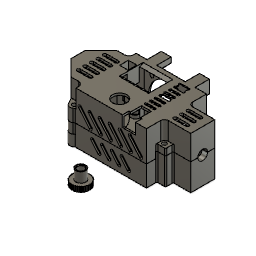
Case_Car_Bat_Mount_Spot Welder_V3 (Autodesk Fusion 360 design; units mm, degrees)
Autodesk Fusion 360 part; units mm, degrees
(part 1 of 5)
sketch "Skizze1" plane through (0, 0, 0) normal (0, 1, 0) x (1, 0, 0)
  circle A0 centre (-27, 22) radius 1.9
  line L0 (1.75, 0) -> (22.5, 0)
  line L1 (0, -1.75) -> (0, -22.5)
  circle A1 centre (27, 22) radius 1.9
  circle A2 centre (-27, -22) radius 1.9
  circle A3 centre (27, -22) radius 1.9
  line L2 (-32.5, 27.5) -> (32.5, 27.5)
  line L3 (32.5, 27.5) -> (32.5, -27.5)
  line L4 (32.5, -27.5) -> (-32.5, -27.5)
  line L5 (-32.5, -27.5) -> (-32.5, 27.5)
  line L6 (-32.5, 27.5) -> (32.5, -27.5) construction
  line L7 (32.5, 27.5) -> (-32.5, -27.5) construction
  point P0 (51.5, 9.5)
  dimension "d3" = 3.8
  dimension "d9" = 22
  dimension "d10" = 27
  dimension "d11" = 65
  dimension "d12" = 55
  constraint symmetric A0 L1 A1
  constraint symmetric A0 L0 A2
  constraint symmetric L0 A1 A3
  constraint perpendicular L2 L3
  constraint parallel L2 L4
  constraint parallel L3 L5
  constraint horizontal L2
  constraint coincident L6 origin
  constraint coincident L7 origin
  measures "d3" diameter of A0
  measures "d9" distance of A0.centre L0
  measures "d10" distance of A0.centre L1
  measures "d11" distance of L3.end L4.end
  measures "d12" distance of L2.end L3.end
extrude "Extrusion1" add sketch "Skizze1" along normal blind 3 makes body 1
sketch "Skizze2" plane through (0, 0, 0) normal (0, -1, 0) x (1, 0, 0)
  circle A0 centre (-27, 22) radius 1.9
  circle A1 centre (-27, -22) radius 1.9
  circle A2 centre (27, 22) radius 1.9
  circle A3 centre (27, -22) radius 1.9
  line L0 (32.5, 27.5) -> (-32.5, 27.5)
  line L1 (-32.5, 27.5) -> (-32.5, -27.5)
  line L2 (-32.5, -27.5) -> (32.5, -27.5)
  line L3 (32.5, -27.5) -> (32.5, 27.5)
  circle A4 centre (-27, 22) radius 1.9
  circle A5 centre (-27, -22) radius 1.9
  circle A6 centre (27, 22) radius 1.9
  circle A7 centre (27, -22) radius 1.9
  line L4 (-32.5, 27.5) -> (32.5, 27.5)
  line L5 (32.5, 27.5) -> (32.5, -27.5)
  line L6 (32.5, -27.5) -> (-32.5, -27.5)
  line L7 (-32.5, -27.5) -> (-32.5, 27.5)
extrude "Extrusion2" add sketch "Skizze2" against normal blind 1.5 contours A0 A4 | A1 A5 | A2 A6 | A3 A7 bodies 1
sketch "Skizze3" plane through (0, 3, 0) normal (0, 1, 0) x (-1, 0, 0)
  circle A0 centre (27, 22) radius 1.9
  circle A1 centre (27, -22) radius 1.9
  circle A2 centre (-27, 22) radius 1.9
  circle A3 centre (-27, -22) radius 1.9
  line L0 (32.5, 27.5) -> (-32.5, 27.5)
  line L1 (-32.5, 27.5) -> (-32.5, -27.5)
  line L2 (-32.5, -27.5) -> (32.5, -27.5)
  line L3 (32.5, -27.5) -> (32.5, 27.5)
  circle A4 centre (27, -22) radius 4
  circle A5 centre (-27, -22) radius 4
  circle A6 centre (27, 22) radius 4
  circle A7 centre (-27, 22) radius 4
  dimension "d17" = 8
  dimension "d18" = 8
  dimension "d19" = 8
  dimension "d20" = 8
  constraint concentric A1 A4
  constraint concentric A3 A5
  constraint concentric A0 A6
  constraint concentric A2 A7
  measures "d17" diameter of A4
  measures "d18" diameter of A6
  measures "d19" diameter of A7
  measures "d20" diameter of A5
extrude "Extrusion3" add sketch "Skizze3" along normal blind 3 contours A4 | A5 | A6 | A7 bodies 1
sketch "Skizze4" plane through (0, 6, 0) normal (0, 1, 0) x (-1, 0, 0)
  circle A0 centre (27, -22) radius 1.9
  circle A1 centre (27, -22) radius 4
  circle A2 centre (27, -22) radius 3
  circle A3 centre (-27, -22) radius 1.9
  circle A4 centre (-27, 22) radius 1.9
  circle A5 centre (27, 22) radius 1.9
  circle A6 centre (-27, -22) radius 3
  circle A7 centre (-27, 22) radius 3
  circle A8 centre (27, 22) radius 3
  dimension "d23" = 6
  dimension "d24" = 6
  dimension "d25" = 6
  dimension "d26" = 6
  constraint concentric A0 A2
  constraint concentric A3 A6
  constraint concentric A4 A7
  constraint concentric A5 A8
  measures "d23" diameter of A2
  measures "d24" diameter of A8
  measures "d25" diameter of A7
  measures "d26" diameter of A6
extrude "Extrusion4" add sketch "Skizze4" along normal blind 4 contours A2 | A6 | A7 | A8 bodies 1
sketch "Skizze5" plane through (0, 0, 0) normal (0, -1, 0) x (1, 0, 0)
  line L0 (32.5, 27.5) -> (-32.5, 27.5)
  line L1 (-32.5, 27.5) -> (-32.5, -27.5)
  line L2 (-32.5, -27.5) -> (32.5, -27.5)
  line L3 (32.5, -27.5) -> (32.5, 27.5)
  line L4 (32.5, -11) -> (56.5, -11)
  line L5 (56.5, -11) -> (56.5, 11)
  line L6 (56.5, 11) -> (32.5, 11)
  line L7 (32.5, 11) -> (32.5, -11)
  line L8 (1.75, 0) -> (22.5, 0)
  dimension "d29" = 24
  dimension "d31" = 22
  constraint horizontal L4
  constraint vertical L5
  constraint horizontal L6
  constraint vertical L7
  constraint coincident L3 L4.start
  constraint symmetric L4 L6 L8
  measures "d29" distance of L4.start L4.end
  measures "d31" vertical distance of L4.end L5.end
extrude "Extrusion5" add sketch "Skizze5" against normal blind 3 contours L3 L4 L5 L6 L7 bodies 1
sketch "Skizze6" plane through (0, 0, 0) normal (0, -1, 0) x (1, 0, 0)
  line L0 (32.5, 27.5) -> (-32.5, 27.5)
  line L1 (-32.5, 27.5) -> (-32.5, -27.5)
  line L2 (-32.5, -27.5) -> (32.5, -27.5)
  line L3 (32.5, -27.5) -> (32.5, -11)
  line L4 (32.5, -11) -> (56.5, -11)
  line L5 (56.5, -11) -> (56.5, 11)
  line L6 (56.5, 11) -> (32.5, 11)
  line L7 (32.5, 11) -> (32.5, 27.5)
  line L8 (-32.5, -21.5) -> (-42.5, -21.5)
  line L9 (-42.5, -21.5) -> (-42.5, 21.5)
  line L10 (-42.5, 21.5) -> (-32.5, 21.5)
  line L11 (-32.5, 21.5) -> (-32.5, -21.5)
  line L12 (1.75, 0) -> (22.5, 0)
  line L13 (-42.5, -21.5) -> (-57.5, -6.5)
  line L14 (-42.5, -21.5) -> (-24.6723, -21.5) construction
  line L15 (-42.5, 21.5) -> (-57.5, 6.5)
  line L16 (-42.5, 21.5) -> (-24.5, 21.5) construction
  line L17 (-57.5, 6.5) -> (-57.5, -6.5)
  dimension "d34" = 10
  dimension "d35" = 43
  dimension "d36" = 135
  dimension "d37" = 135
  dimension "d38" = 15
  constraint horizontal L8
  constraint vertical L9
  constraint horizontal L10
  constraint vertical L11
  constraint coincident L1 L8.start
  constraint symmetric L8 L10 L12
  constraint horizontal L14
  constraint horizontal L16
  constraint parallel L9 L17
  measures "d34" distance of L8.start L8.end
  measures "d35" distance of L8.start L10.end
  measures "d36" angle of L13 L14
  measures "d37" angle of L15 L16
  measures "d38" distance of L9 L17
extrude "Extrusion6" add sketch "Skizze6" against normal blind 3 contours L1 L8 L9 L10 L11 | L9 L13 L15 L17 bodies 1
sketch "Skizze7" plane through (0, 3, 0) normal (0, 1, 0) x (-1, 0, 0)
  circle A0 centre (-27, -22) radius 4
  circle A1 centre (27, -22) radius 4
  circle A2 centre (-27, 22) radius 4
  circle A3 centre (27, 22) radius 4
  line L0 (32.5, 27.5) -> (-32.5, 27.5)
  line L1 (-32.5, 27.5) -> (-32.5, 11)
  line L2 (-32.5, 11) -> (-56.5, 11)
  line L3 (-56.5, 11) -> (-56.5, -11)
  line L4 (-56.5, -11) -> (-32.5, -11)
  line L5 (-32.5, -11) -> (-32.5, -27.5)
  line L6 (-32.5, -27.5) -> (32.5, -27.5)
  line L7 (32.5, -27.5) -> (32.5, -21.5)
  line L8 (32.5, -21.5) -> (42.5, -21.5)
  line L9 (42.5, -21.5) -> (57.5, -6.5)
  line L10 (57.5, -6.5) -> (57.5, 6.5)
  line L11 (57.5, 6.5) -> (42.5, 21.5)
  line L12 (42.5, 21.5) -> (32.5, 21.5)
  line L13 (32.5, 21.5) -> (32.5, 27.5)
  line L14 (32.5, -27.5) -> (32.5, -21.5)
  line L15 (-32.5, -27.5) -> (32.5, -27.5)
  line L16 (32.5, -21.5) -> (42.5, -21.5)
  line L17 (42.5, -21.5) -> (57.5, -6.5)
  line L18 (57.5, -6.5) -> (57.5, 6.5)
  line L19 (57.5, 6.5) -> (42.5, 21.5)
  line L20 (42.5, 21.5) -> (32.5, 21.5)
  line L21 (32.5, 21.5) -> (32.5, 27.5)
  line L22 (32.5, 27.5) -> (-32.5, 27.5)
  line L23 (-32.5, 27.5) -> (-32.5, 11)
  line L24 (-32.5, 11) -> (-56.5, 11)
  line L25 (-32.5, 27.5) -> (32.5, 27.5)
  line L26 (32.5, 27.5) -> (32.5, 21.5)
  line L27 (32.5, 21.5) -> (42.5, 21.5)
  line L28 (42.5, 21.5) -> (57.5, 6.5)
  line L29 (57.5, 6.5) -> (57.5, -6.5)
  line L30 (57.5, -6.5) -> (42.5, -21.5)
  line L31 (42.5, -21.5) -> (32.5, -21.5)
  line L32 (32.5, -21.5) -> (32.5, -27.5)
  line L33 (32.5, -27.5) -> (-32.5, -27.5)
  line L34 (-32.5, -27.5) -> (-32.5, -11)
  line L35 (-32.5, -11) -> (-56.5, -11)
  line L36 (-56.5, -11) -> (-56.5, 11)
  line L37 (-56.5, 11) -> (-32.5, 11)
  line L38 (-32.5, 11) -> (-32.5, 27.5)
  line L39 (31, -26) -> (-31, -26)
  line L40 (-31, -26) -> (-31, -9.8787)
  line L41 (-31, -9.8787) -> (-31, -9.5)
  line L42 (-31, -9.5) -> (-55, -9.5)
  line L43 (-55, -9.5) -> (-55, 9.5)
  line L44 (-55, 9.5) -> (-31, 9.5)
  line L45 (-31, 9.5) -> (-31, 26)
  line L46 (-31, 26) -> (31, 26)
  line L47 (31, 26) -> (31, 20)
  line L48 (31, 20) -> (41.8787, 20)
  line L49 (41.8787, 20) -> (56, 5.8787)
  line L50 (56, 5.8787) -> (56, -5.8787)
  line L51 (56, -5.8787) -> (41.8787, -20)
  line L52 (41.8787, -20) -> (31, -20)
  line L53 (31, -20) -> (31, -26)
  dimension "d41" = 1.5
  dimension "d42" = 1.5
  dimension "d43" = 1.5
  dimension "d44" = 1.5
  dimension "d45" = 1.5
  dimension "d46" = 1.5
  dimension "d47" = 1.5
  dimension "d48" = 1.5
  dimension "d49" = 1.5
  dimension "d50" = 1.5
  dimension "d51" = 1.5
  dimension "d52" = 1.5
  dimension "d53" = 1.5
  dimension "d54" = 1.5
  constraint perpendicular L7 L39
  constraint perpendicular L35 L40
  constraint perpendicular L35 L41
  constraint perpendicular L40 L42
  constraint perpendicular L42 L43
  constraint perpendicular L43 L44
  constraint perpendicular L44 L45
  constraint perpendicular L26 L46
  constraint perpendicular L46 L47
  constraint perpendicular L47 L48
  constraint perpendicular L46 L50
  constraint perpendicular L50 L52
  constraint perpendicular L39 L53
  constraint parallel L9 L51
  constraint parallel L11 L49
  measures "d41" distance of L10 L50
  measures "d42" distance of L9 L51
  measures "d43" distance of L8 L52
  measures "d44" distance of L7 L53
  measures "d45" distance of L6 L39
  measures "d46" distance of L5 L40
  measures "d47" distance of L4 L42
  measures "d48" distance of L3 L43
  measures "d49" distance of L2 L44
  measures "d50" distance of L1 L45
  measures "d51" distance of L0 L46
  measures "d52" distance of L13 L47
  measures "d53" distance of L12 L48
  measures "d54" distance of L11 L49
extrude "Extrusion7" add sketch "Skizze7" along normal blind 13 bodies 1
sketch "Skizze8" plane through (0, 3, 0) normal (0, 1, 0) x (-1, 0, 0)
  line L0 (51.5218, -10.3569) -> (51.5218, 10.3569)
  line L1 (-31, -9.5) -> (-31, -22)
  line L2 (-31, 22) -> (-31, 9.5)
  line L3 (-31, 9.5) -> (-55, 9.5)
  line L4 (-55, 9.5) -> (-55, -9.5)
  line L5 (-55, -9.5) -> (-31, -9.5)
  line L6 (-27, -26) -> (27, -26)
  arc A0 (31, -22) -> (27, -26) centre (27, -22) ccw
  line L7 (31, -22) -> (31, -20)
  line L8 (31, -20) -> (41.8787, -20)
  line L9 (41.8787, -20) -> (56, -5.8787)
  line L10 (56, -5.8787) -> (56, 5.8787)
  line L11 (56, 5.8787) -> (41.8787, 20)
  line L12 (41.8787, 20) -> (31, 20)
  line L13 (31, 20) -> (31, 22)
  arc A1 (27, 26) -> (31, 22) centre (27, 22) ccw
  arc A2 (-31, 22) -> (-27, 26) centre (-27, 22) ccw
  line L14 (27, 26) -> (-27, 26)
  arc A3 (-27, -26) -> (-31, -22) centre (-27, -22) ccw
  constraint coincident L0.end L11
  constraint coincident L0.start L9
  constraint parallel L0 L10
extrude "Extrusion8" add sketch "Skizze8" along normal up to surface (13 mm away) contours L0 L9 L10 L11 bodies 1
sketch "Skizze9" plane through (-57.5, 0, 0) normal (-1, 0, 0) x (0, 0, 1)
  line L0 (-6.5, 0) -> (6.5, 0)
  line L1 (6.5, 0) -> (6.5, 16)
  line L2 (6.5, 16) -> (-6.5, 16)
  line L3 (-6.5, 16) -> (-6.5, 0)
  line L4 (0, 1.75) -> (0, 22.5)
  line L5 (-6.5, 16) -> (6.5, 16)
  circle A0 centre (0, 16) radius 5
  dimension "d60" = 10
  constraint midpoint L5 A0.centre
  measures "d60" diameter of A0
extrude "Extrusion9" cut sketch "Skizze9" against normal blind 6 contours L2 L4 L5 A0 | L2 L4 L5 A0 picked at (-3.3164, 15.7628) picked at (2.6617, 14.0075) bodies 1
sketch "Skizze12" plane through (0, 3, 0) normal (0, 1, 0) x (-1, 0, 0)
  line L0 (51.5218, -10.3569) -> (51.5218, 10.3569)
  line L1 (51.5218, 10.3569) -> (41.8787, 20)
  line L2 (41.8787, 20) -> (31, 20)
  line L3 (31, 20) -> (31, 22)
  arc A0 (27, 26) -> (31, 22) centre (27, 22) ccw
  arc A1 (-31, 22) -> (-27, 26) centre (-27, 22) ccw
  line L4 (-31, 22) -> (-31, 9.5)
  line L5 (-31, 9.5) -> (-55, 9.5)
  line L6 (-55, 9.5) -> (-55, -9.5)
  line L7 (-55, -9.5) -> (-31, -9.5)
  arc A2 (-27, -26) -> (-31, -22) centre (-27, -22) ccw
  arc A3 (31, -22) -> (27, -26) centre (27, -22) ccw
  line L8 (31, -22) -> (31, -20)
  line L9 (31, -20) -> (41.8787, -20)
  line L10 (41.8787, -20) -> (51.5218, -10.3569)
  line L11 (-51.5, 9.5) -> (-51.5, -9.5)
  line L12 (-31, -9.5) -> (-31, -22)
  line L13 (-27, -26) -> (27, -26)
  line L14 (27, 26) -> (-27, 26)
  constraint coincident L5 L11.start
  constraint coincident L7 L11.end
  constraint parallel L6 L11
extrude "Extrusion12" add sketch "Skizze12" along normal blind 13 contours L5 L6 L7 L11 bodies 1
sketch "Skizze16" plane through (0, 6, 0) normal (0, 1, 0) x (-1, 0, 0)
  circle A0 centre (27, -22) radius 3
  line L0 (-51.5, 9.5) -> (-51.5, -9.5)
  line L1 (-51.5, -9.5) -> (-31, -9.5)
  line L2 (-31, -9.5) -> (-31, -22)
  arc A1 (-27, -26) -> (-31, -22) centre (-27, -22) ccw
  line L3 (-27, -26) -> (27, -26)
  arc A2 (31, -22) -> (27, -26) centre (27, -22) ccw
  line L4 (31, -22) -> (31, -20)
  line L5 (31, -20) -> (41.8787, -20)
  line L6 (41.8787, -20) -> (51.5218, -10.3569)
  line L7 (51.5218, -10.3569) -> (51.5218, 10.3569)
  line L8 (51.5218, 10.3569) -> (41.8787, 20)
  line L9 (41.8787, 20) -> (31, 20)
  line L10 (31, 20) -> (31, 22)
  arc A3 (27, 26) -> (31, 22) centre (27, 22) ccw
  line L11 (27, 26) -> (-27, 26)
  arc A4 (-31, 22) -> (-27, 26) centre (-27, 22) ccw
  line L12 (-31, 22) -> (-31, 9.5)
  line L13 (-31, 9.5) -> (-51.5, 9.5)
  line L14 (31, -22) -> (23, -22)
  line L15 (23, -22) -> (23, -26)
  line L16 (23, -26) -> (31, -26)
  line L17 (31, -26) -> (31, -22)
  line L18 (-31, -26) -> (-23, -26)
  line L19 (-23, -26) -> (-23, -22)
  line L20 (-23, -22) -> (-31, -22)
  line L21 (-31, -22) -> (-31, -26)
  line L22 (-31, 22) -> (-23, 22)
  line L23 (-23, 22) -> (-23, 26)
  line L24 (-23, 26) -> (-31, 26)
  line L25 (-31, 26) -> (-31, 22)
  line L26 (31, 22) -> (23, 22)
  line L27 (23, 22) -> (23, 26)
  line L28 (23, 26) -> (31, 26)
  line L29 (31, 26) -> (31, 22)
  circle A5 centre (27, 22) radius 1.9
  circle A6 centre (27, 22) radius 3
  circle A7 centre (27, -22) radius 1.9
  circle A8 centre (27, -22) radius 1.9
  circle A9 centre (27, -22) radius 3
  circle A10 centre (-27, -22) radius 1.9
  circle A11 centre (-27, -22) radius 3
  circle A12 centre (-27, 22) radius 1.9
  circle A13 centre (-27, 22) radius 3
  arc A14 (31, -22) -> (27, -26) centre (27, -22) ccw
  arc A15 (27, -26) -> (31, -22) centre (27, -22) ccw
  point P0 (-31, -26)
  dimension "d76" = 4
  dimension "d77" = 8
  dimension "d78" = 8
  dimension "d79" = 8
  constraint horizontal L14
  constraint vertical L15
  constraint horizontal L16
  constraint vertical L17
  constraint coincident A2.start L4.start
  constraint horizontal L18
  constraint vertical L19
  constraint horizontal L20
  constraint vertical L21
  constraint coincident P0 L18.start
  constraint horizontal L22
  constraint vertical L23
  constraint horizontal L24
  constraint vertical L25
  constraint coincident A4.start L12.start
  constraint horizontal L26
  constraint vertical L27
  constraint horizontal L28
  constraint vertical L29
  constraint coincident L10.end A3.end
  measures "d76" distance of P0 L2.end
  measures "d77" distance of P0 L18.end
  measures "d78" distance of A4.start L22.end
  measures "d79" distance of L10.end L26.end
extrude "Extrusion15" add sketch "Skizze16" along normal blind 4 and the other way blind 3 contours A0 A2 L14 A9 A14 A15 | L16 L17 A15 | L3 A2 L15 L16 A14 | A1 L3 L18 L19 | A1 L18 L20 L21 A11 | A3 L26 L28 L29 A6 | A3 L11 L27 L28 | A4 L22 L24 L25 A13 | L11 A4 L23 L24 bodies 1
sketch "Skizze18" plane through (0, 3, 0) normal (0, 1, 0) x (-1, 0, 0)
  line L0 (-23, 26) -> (-23, 22)
  arc A0 (-31, 22) -> (-23, 22) centre (-27, 22) ccw
  line L1 (-31, 22) -> (-31, 9.5)
  line L2 (-31, 9.5) -> (-51.5, 9.5)
  line L3 (-51.5, 9.5) -> (-51.5, -9.5)
  line L4 (-51.5, -9.5) -> (-31, -9.5)
  line L5 (-31, -9.5) -> (-31, -22)
  arc A1 (-23, -22) -> (-31, -22) centre (-27, -22) ccw
  line L6 (-23, -22) -> (-23, -26)
  line L7 (-23, -26) -> (23, -26)
  line L8 (23, -26) -> (23, -22)
  arc A2 (31, -22) -> (23, -22) centre (27, -22) ccw
  line L9 (31, -22) -> (31, -20)
  line L10 (31, -20) -> (41.8787, -20)
  line L11 (41.8787, -20) -> (51.5218, -10.3569)
  line L12 (51.5218, -10.3569) -> (51.5218, 10.3569)
  line L13 (51.5218, 10.3569) -> (41.8787, 20)
  line L14 (41.8787, 20) -> (31, 20)
  line L15 (31, 20) -> (31, 22)
  arc A3 (23, 22) -> (31, 22) centre (27, 22) ccw
  line L16 (23, 22) -> (23, 26)
  line L17 (23, 26) -> (-23, 26)
  circle A4 centre (36, 25) radius 3.5
  line L18 (32.5, 21.5) -> (32.5, 27.5)
  line L19 (42.5, 21.5) -> (32.5, 21.5)
  circle A5 centre (36, 25) radius 1.9
  line L20 (42.5, 21.5) -> (38.922, 26.9266)
  line L21 (32.5, 27.5) -> (34.8649, 28.3108)
  line L22 (-1.75, 0) -> (-22.5, 0)
  line L23 (42.5, -21.5) -> (38.922, -26.9266)
  circle A6 centre (36, -25) radius 3.5
  line L24 (32.5, -27.5) -> (34.8649, -28.3108)
  circle A7 centre (36, -25) radius 1.9
  line L25 (42.5, -21.5) -> (32.5, -21.5)
  line L26 (32.5, -21.5) -> (32.5, -27.5)
  dimension "d89" = 7
  dimension "d90" = 3.8
  constraint tangent A4 L18
  constraint tangent A4 L19
  constraint concentric A4 A5
  constraint coincident L19.start L20.start
  constraint coincident A4 L20.end
  constraint tangent A4 L20
  constraint coincident L18.end L21.start
  constraint coincident A4 L21.end
  constraint tangent A4 L21
  constraint symmetric A4 L22 A6
  constraint symmetric L18.start L22 L25.end
  constraint symmetric L18.end L22 L24.start
  constraint symmetric L19.start L22 L23.start
  constraint symmetric A5 L22 A7
  constraint symmetric L20.end L22 L23.end
  constraint symmetric L21.end L22 L24.end
  measures "d89" diameter of A4
  measures "d90" diameter of A5
extrude "Extrusion16" add sketch "Skizze18" along normal blind 13 and the other way blind 3 contours A4 | A4 L19 L20 | A4 L18 L19 | A4 L18 L21 | L23 A6 L25 | A6 | A6 L25 L26 | A6 L24 L26 bodies 1
sketch "Skizze19" plane through (0, 3, 0) normal (0, 1, 0) x (-1, 0, 0)
  line L0 (-23, 26) -> (-23, 22)
  arc A0 (-31, 22) -> (-23, 22) centre (-27, 22) ccw
  line L1 (-31, 22) -> (-31, 9.5)
  line L2 (-31, 9.5) -> (-51.5, 9.5)
  line L3 (-51.5, 9.5) -> (-51.5, -9.5)
  line L4 (-51.5, -9.5) -> (-31, -9.5)
  line L5 (-31, -9.5) -> (-31, -22)
  arc A1 (-23, -22) -> (-31, -22) centre (-27, -22) ccw
  line L6 (-23, -22) -> (-23, -26)
  line L7 (-23, -26) -> (23, -26)
  line L8 (23, -26) -> (23, -22)
  arc A2 (31, -22) -> (23, -22) centre (27, -22) ccw
  line L9 (31, -22) -> (31, -20)
  line L10 (31, -20) -> (41.8787, -20)
  line L11 (41.8787, -20) -> (51.5218, -10.3569)
  line L12 (51.5218, -10.3569) -> (51.5218, 10.3569)
  line L13 (51.5218, 10.3569) -> (41.8787, 20)
  line L14 (41.8787, 20) -> (31, 20)
  line L15 (31, 20) -> (31, 22)
  arc A3 (23, 22) -> (31, 22) centre (27, 22) ccw
  line L16 (23, 22) -> (23, 26)
  line L17 (23, 26) -> (-23, 26)
  line L18 (-32.5, 11) -> (-39.5, 11)
  line L19 (-39.5, 11) -> (-39.5, 18)
  line L20 (-39.5, 18) -> (-32.5, 18)
  line L21 (-32.5, 18) -> (-32.5, 11)
  circle A4 centre (-36, 14.5) radius 1.9
  line L22 (-1.75, 0) -> (-22.5, 0)
  line L23 (-39.5, -11) -> (-39.5, -18)
  line L24 (-39.5, -18) -> (-32.5, -18)
  circle A5 centre (-36, -14.5) radius 1.9
  line L25 (-32.5, -11) -> (-32.5, -27.5)
  line L26 (-56.5, -11) -> (-32.5, -11)
  point P0 (-32.5, 11)
  dimension "d95" = 7
  dimension "d96" = 7
  dimension "d97" = 3.8
  dimension "d98" = 3.5
  dimension "d99" = 3.5
  constraint horizontal L18
  constraint vertical L19
  constraint horizontal L20
  constraint vertical L21
  constraint coincident P0 L18.start
  constraint symmetric L18.end L22 L23.start
  constraint symmetric L19.end L22 L23.end
  constraint symmetric L20.end L22 L24.end
  constraint symmetric A4 L22 A5
  measures "d95" distance of P0 L18.end
  measures "d96" distance of P0 L20.end
  measures "d97" diameter of A4
  measures "d98" distance of L18 A4.centre
  measures "d99" distance of L21 A4.centre
extrude "Extrusion17" add sketch "Skizze19" along normal blind 13 and the other way blind 3 contours L18 L19 L20 L21 | L23 L24 L25 L26 bodies 1
fillet "Abrundung1" radius 1 6 edges at (32.5, 8, 18) (39.5, 8, 11) (39.5, 8, -11) (32.5, 8, -18) (39.5, 8, 18) (39.5, 8, -18) on bodies 1
sketch "Skizze20" plane through (0, 16, 0) normal (0, 1, 0) x (-1, 0, 0)
  arc A0 (-39.5, -17) -> (-38.5, -18) centre (-38.5, -17) ccw
  line L0 (-38.5, -18) -> (-33.5, -18)
  arc A1 (-32.5, -19) -> (-33.5, -18) centre (-33.5, -19) ccw
  line L1 (-32.5, -19) -> (-32.5, -27.5)
  line L2 (-32.5, -27.5) -> (32.5, -27.5)
  line L3 (32.5, -27.5) -> (34.8649, -28.3108)
  arc A2 (34.8649, -28.3108) -> (38.922, -26.9266) centre (36, -25) ccw
  line L4 (38.922, -26.9266) -> (42.5, -21.5)
  line L5 (42.5, -21.5) -> (57.5, -6.5)
  line L6 (57.5, -6.5) -> (57.5, -5)
  line L7 (57.5, -5) -> (51.5218, -5)
  line L8 (51.5218, -5) -> (51.5218, -10.3569)
  line L9 (51.5218, -10.3569) -> (41.8787, -20)
  line L10 (41.8787, -20) -> (31, -20)
  line L11 (31, -20) -> (31, -26)
  line L12 (31, -26) -> (-31, -26)
  line L13 (-31, -26) -> (-31, -9.5)
  line L14 (-31, -9.5) -> (-51.5, -9.5)
  line L15 (-51.5, -9.5) -> (-51.5, 9.5)
  line L16 (-51.5, 9.5) -> (-31, 9.5)
  line L17 (-31, 9.5) -> (-31, 26)
  line L18 (-31, 26) -> (31, 26)
  line L19 (31, 26) -> (31, 20)
  line L20 (31, 20) -> (41.8787, 20)
  line L21 (41.8787, 20) -> (51.5218, 10.3569)
  line L22 (51.5218, 10.3569) -> (51.5218, 5)
  line L23 (51.5218, 5) -> (57.5, 5)
  line L24 (57.5, 5) -> (57.5, 6.5)
  line L25 (57.5, 6.5) -> (42.5, 21.5)
  line L26 (42.5, 21.5) -> (38.922, 26.9266)
  arc A3 (38.922, 26.9266) -> (34.8649, 28.3108) centre (36, 25) ccw
  line L27 (34.8649, 28.3108) -> (32.5, 27.5)
  line L28 (32.5, 27.5) -> (-32.5, 27.5)
  line L29 (-32.5, 27.5) -> (-32.5, 19)
  arc A4 (-33.5, 18) -> (-32.5, 19) centre (-33.5, 19) ccw
  line L30 (-33.5, 18) -> (-38.5, 18)
  arc A5 (-38.5, 18) -> (-39.5, 17) centre (-38.5, 17) ccw
  line L31 (-39.5, 17) -> (-39.5, 12)
  arc A6 (-40.5, 11) -> (-39.5, 12) centre (-40.5, 12) ccw
  line L32 (-40.5, 11) -> (-56.5, 11)
  line L33 (-56.5, 11) -> (-56.5, -11)
  line L34 (-56.5, -11) -> (-40.5, -11)
  arc A7 (-39.5, -12) -> (-40.5, -11) centre (-40.5, -12) ccw
  line L35 (-39.5, -12) -> (-39.5, -17)
  circle A8 centre (-36, 14.5) radius 1.9
  circle A9 centre (-36, -14.5) radius 1.9
  circle A10 centre (36, -25) radius 1.9
  circle A11 centre (36, 25) radius 1.9
  circle A12 centre (-36, 14.5) radius 1.9
  circle A13 centre (-36, -14.5) radius 1.9
  circle A14 centre (36, -25) radius 1.9
  circle A15 centre (36, 25) radius 1.9
  arc A16 (-39.5, -17) -> (-38.5, -18) centre (-38.5, -17) ccw
  line L36 (-39.5, -17) -> (-39.5, -12)
  arc A17 (-39.5, -12) -> (-40.5, -11) centre (-40.5, -12) ccw
  line L37 (-40.5, -11) -> (-56.5, -11)
  line L38 (-56.5, -11) -> (-56.5, 11)
  line L39 (-56.5, 11) -> (-40.5, 11)
  arc A18 (-40.5, 11) -> (-39.5, 12) centre (-40.5, 12) ccw
  line L40 (-39.5, 12) -> (-39.5, 17)
  arc A19 (-38.5, 18) -> (-39.5, 17) centre (-38.5, 17) ccw
  line L41 (-38.5, 18) -> (-33.5, 18)
  arc A20 (-33.5, 18) -> (-32.5, 19) centre (-33.5, 19) ccw
  line L42 (-32.5, 19) -> (-32.5, 27.5)
  line L43 (-32.5, 27.5) -> (32.5, 27.5)
  line L44 (32.5, 27.5) -> (34.8649, 28.3108)
  arc A21 (38.922, 26.9266) -> (34.8649, 28.3108) centre (36, 25) ccw
  line L45 (38.922, 26.9266) -> (42.5, 21.5)
  line L46 (42.5, 21.5) -> (57.5, 6.5)
  line L47 (57.5, 6.5) -> (57.5, -6.5)
  line L48 (57.5, -6.5) -> (42.5, -21.5)
  line L49 (42.5, -21.5) -> (38.922, -26.9266)
  arc A22 (34.8649, -28.3108) -> (38.922, -26.9266) centre (36, -25) ccw
  line L50 (34.8649, -28.3108) -> (32.5, -27.5)
  line L51 (32.5, -27.5) -> (-32.5, -27.5)
  line L52 (-32.5, -27.5) -> (-32.5, -19)
  arc A23 (-32.5, -19) -> (-33.5, -18) centre (-33.5, -19) ccw
  line L53 (-33.5, -18) -> (-38.5, -18)
  line L54 (-51.5, -9.5) -> (-51.5, 9.5)
  line L55 (-51.5, 9.5) -> (-31, 9.5)
  line L56 (-23, 26) -> (-23, 22)
  arc A24 (-31, 22) -> (-23, 22) centre (-27, 22) ccw
  line L57 (-31, 22) -> (-31, 9.5)
  line L58 (-31, 9.5) -> (-51.5, 9.5)
  line L59 (-51.5, 9.5) -> (-51.5, -9.5)
  line L60 (-51.5, -9.5) -> (-31, -9.5)
  line L61 (-31, -9.5) -> (-31, -22)
  arc A25 (-23, -22) -> (-31, -22) centre (-27, -22) ccw
  line L62 (-23, -22) -> (-23, -26)
  line L63 (-23, -26) -> (23, -26)
  line L64 (23, -26) -> (23, -22)
  arc A26 (31, -22) -> (23, -22) centre (27, -22) ccw
  line L65 (31, -22) -> (31, -20)
  line L66 (31, -20) -> (41.8787, -20)
  line L67 (41.8787, -20) -> (51.5218, -10.3569)
  line L68 (51.5218, -10.3569) -> (51.5218, 10.3569)
  line L69 (51.5218, 10.3569) -> (41.8787, 20)
  line L70 (41.8787, 20) -> (31, 20)
  line L71 (31, 20) -> (31, 22)
  arc A27 (23, 22) -> (31, 22) centre (27, 22) ccw
  line L72 (23, 22) -> (23, 26)
  line L73 (23, 26) -> (-23, 26)
  line L74 (-32.5, 19) -> (-31, 19)
  line L75 (-32.5, -19) -> (-31, -19)
  constraint coincident L29.end A4.end
  constraint coincident L57 L74.end
  constraint coincident A1.start L1.start
  constraint coincident L61 L75.end
extrude "Extrusion18" add sketch "Skizze20" along normal blind 5.5 contours A0 L0 A1 L13 L14 L15 L16 L17 A4 L30 A5 L31 A6 L32 L33 L34 A7 L35 A16 L36 A17 L37 L38 L39 A18 L40 A19 L41 A20 A23 L53 L54 L55 L57 L58 L59 L60 L61 L74 L75 bodies 1
sketch "Skizze21" plane through (56.5, 0, 0) normal (1, 0, 0) x (0, 0, -1)
  line L0 (-11, 0) -> (11, 0)
  line L1 (11, 0) -> (11, 21.5)
  line L2 (11, 21.5) -> (-11, 21.5)
  line L3 (-11, 21.5) -> (-11, 0)
  circle A0 centre (0, 21.5) radius 5
  dimension "d107" = 10
  constraint midpoint L2 A0.centre
  measures "d107" diameter of A0
extrude "Extrusion19" cut sketch "Skizze21" against normal blind 5 contours L2 A0 picked at (-1.6112, 20.7603) bodies 1
sketch "Skizze22" plane through (0, 21.5, 0) normal (0, 1, 0) x (-1, 0, 0)
  line L0 (-56.5, 5) -> (-51.5, 5)
  line L1 (-51.5, 5) -> (-51.5, 9.5)
  line L2 (-51.5, 9.5) -> (-31, 9.5)
  line L3 (-31, 9.5) -> (-31, 19)
  line L4 (-31, 19) -> (-32.5, 19)
  arc A0 (-33.5, 18) -> (-32.5, 19) centre (-33.5, 19) ccw
  line L5 (-33.5, 18) -> (-38.5, 18)
  arc A1 (-38.5, 18) -> (-39.5, 17) centre (-38.5, 17) ccw
  line L6 (-39.5, 17) -> (-39.5, 12)
  arc A2 (-40.5, 11) -> (-39.5, 12) centre (-40.5, 12) ccw
  line L7 (-40.5, 11) -> (-56.5, 11)
  line L8 (-56.5, 11) -> (-56.5, 5)
  circle A3 centre (-36, 14.5) radius 1.9
  line L9 (-51.5, -5) -> (-56.5, -5)
  line L10 (-56.5, -5) -> (-56.5, -11)
  line L11 (-56.5, -11) -> (-40.5, -11)
  arc A4 (-39.5, -12) -> (-40.5, -11) centre (-40.5, -12) ccw
  line L12 (-39.5, -12) -> (-39.5, -17)
  arc A5 (-39.5, -17) -> (-38.5, -18) centre (-38.5, -17) ccw
  line L13 (-38.5, -18) -> (-33.5, -18)
  arc A6 (-32.5, -19) -> (-33.5, -18) centre (-33.5, -19) ccw
  line L14 (-32.5, -19) -> (-31, -19)
  line L15 (-31, -19) -> (-31, -9.5)
  line L16 (-31, -9.5) -> (-51.5, -9.5)
  line L17 (-51.5, -9.5) -> (-51.5, -5)
  circle A7 centre (-36, -14.5) radius 1.9
  circle A8 centre (-36, 14.5) radius 1.9
  circle A9 centre (-36, -14.5) radius 1.9
  circle A10 centre (36, -25) radius 1.9
  circle A11 centre (36, 25) radius 1.9
  arc A12 (-39.5, -17) -> (-38.5, -18) centre (-38.5, -17) ccw
  line L18 (-39.5, -17) -> (-39.5, -12)
  arc A13 (-39.5, -12) -> (-40.5, -11) centre (-40.5, -12) ccw
  line L19 (-40.5, -11) -> (-56.5, -11)
  line L20 (-56.5, -11) -> (-56.5, 11)
  line L21 (-56.5, 11) -> (-40.5, 11)
  arc A14 (-40.5, 11) -> (-39.5, 12) centre (-40.5, 12) ccw
  line L22 (-39.5, 12) -> (-39.5, 17)
  arc A15 (-38.5, 18) -> (-39.5, 17) centre (-38.5, 17) ccw
  line L23 (-38.5, 18) -> (-33.5, 18)
  arc A16 (-33.5, 18) -> (-32.5, 19) centre (-33.5, 19) ccw
  line L24 (-32.5, 19) -> (-32.5, 27.5)
  line L25 (-32.5, 27.5) -> (32.5, 27.5)
  line L26 (32.5, 27.5) -> (34.8649, 28.3108)
  arc A17 (38.922, 26.9266) -> (34.8649, 28.3108) centre (36, 25) ccw
  line L27 (38.922, 26.9266) -> (42.5, 21.5)
  line L28 (42.5, 21.5) -> (57.5, 6.5)
  line L29 (57.5, 6.5) -> (57.5, -6.5)
  line L30 (57.5, -6.5) -> (42.5, -21.5)
  line L31 (42.5, -21.5) -> (38.922, -26.9266)
  arc A18 (34.8649, -28.3108) -> (38.922, -26.9266) centre (36, -25) ccw
  line L32 (34.8649, -28.3108) -> (32.5, -27.5)
  line L33 (32.5, -27.5) -> (-32.5, -27.5)
  line L34 (-32.5, -27.5) -> (-32.5, -19)
  arc A19 (-32.5, -19) -> (-33.5, -18) centre (-33.5, -19) ccw
  line L35 (-33.5, -18) -> (-38.5, -18)
  line L36 (-23, 26) -> (-23, 22)
  arc A20 (-31, 22) -> (-23, 22) centre (-27, 22) ccw
  line L37 (-31, 22) -> (-31, 9.5)
  line L38 (-31, 9.5) -> (-51.5, 9.5)
  line L39 (-51.5, 9.5) -> (-51.5, -9.5)
  line L40 (-51.5, -9.5) -> (-31, -9.5)
  line L41 (-31, -9.5) -> (-31, -22)
  arc A21 (-23, -22) -> (-31, -22) centre (-27, -22) ccw
  line L42 (-23, -22) -> (-23, -26)
  line L43 (-23, -26) -> (23, -26)
  line L44 (23, -26) -> (23, -22)
  arc A22 (31, -22) -> (23, -22) centre (27, -22) ccw
  line L45 (31, -22) -> (31, -20)
  line L46 (31, -20) -> (41.8787, -20)
  line L47 (41.8787, -20) -> (51.5218, -10.3569)
  line L48 (51.5218, -10.3569) -> (51.5218, 10.3569)
  line L49 (51.5218, 10.3569) -> (41.8787, 20)
  line L50 (41.8787, 20) -> (31, 20)
  line L51 (31, 20) -> (31, 22)
  arc A23 (23, 22) -> (31, 22) centre (27, 22) ccw
  line L52 (23, 22) -> (23, 26)
  line L53 (23, 26) -> (-23, 26)
  circle A24 centre (27, -22) radius 1.9
  arc A25 (30, -22) -> (24, -22) centre (27, -22) ccw
  line L54 (24, -22) -> (23, -22)
  line L55 (23, -22) -> (23, -26)
  line L56 (23, -26) -> (31, -26)
  line L57 (31, -26) -> (31, -22)
  line L58 (31, -22) -> (30, -22)
  circle A26 centre (-27, -22) radius 1.9
  arc A27 (-24, -22) -> (-30, -22) centre (-27, -22) ccw
  line L59 (-30, -22) -> (-31, -22)
  line L60 (-31, -22) -> (-31, -26)
  line L61 (-31, -26) -> (-23, -26)
  line L62 (-23, -26) -> (-23, -22)
  line L63 (-23, -22) -> (-24, -22)
  circle A28 centre (-27, 22) radius 1.9
  arc A29 (-30, 22) -> (-24, 22) centre (-27, 22) ccw
  line L64 (-24, 22) -> (-23, 22)
  line L65 (-23, 22) -> (-23, 26)
  line L66 (-23, 26) -> (-31, 26)
  line L67 (-31, 26) -> (-31, 22)
  line L68 (-31, 22) -> (-30, 22)
  circle A30 centre (27, 22) radius 1.9
  arc A31 (24, 22) -> (30, 22) centre (27, 22) ccw
  line L69 (30, 22) -> (31, 22)
  line L70 (31, 22) -> (31, 26)
  line L71 (31, 26) -> (23, 26)
  line L72 (23, 26) -> (23, 22)
  line L73 (23, 22) -> (24, 22)
extrude "Extrusion20" add sketch "Skizze22" along normal blind 23.5 separate body contours L0 L1 L2 L3 L4 A0 L5 A1 L6 A2 L7 L8 L20 L21 A14 L22 A15 L23 A16 L37 L38 L39 | L0 L9 L20 L39 | L9 L10 L11 A4 L12 A5 L13 A6 L14 L15 L16 L17 A12 L18 A13 L19 L20 A19 L35 L39 L40 L41 | L4 L14 L24 L25 L26 A17 L27 L28 L29 L30 L31 A18 L32 L33 L34 L37 L41 L43 L45 L46 L47 L48 L49 L50 L51 L53 L56 L57 L60 L61 L66 L67 L70 L71 makes body 2
sketch "Skizze23" plane through (0, 21.5, 0) normal (0, -1, 0) x (1, 0, 0)
  circle A0 centre (36, 14.5) radius 1.9
  circle A1 centre (-36, 25) radius 1.9
  circle A2 centre (-36, -25) radius 1.9
  line L0 (-31, 26) -> (31, 26)
  line L1 (31, 26) -> (31, 9.5)
  line L2 (31, 9.5) -> (51.5, 9.5)
  line L3 (51.5, 9.5) -> (51.5, -9.5)
  line L4 (51.5, -9.5) -> (31, -9.5)
  line L5 (31, -9.5) -> (31, -26)
  line L6 (31, -26) -> (23, -26)
  line L7 (23, -26) -> (-23, -26)
  line L8 (-23, -26) -> (-31, -26)
  line L9 (-31, -26) -> (-31, -20)
  line L10 (-31, -20) -> (-41.8787, -20)
  line L11 (-41.8787, -20) -> (-51.5218, -10.3569)
  line L12 (-51.5218, -10.3569) -> (-51.5218, 10.3569)
  line L13 (-51.5218, 10.3569) -> (-41.8787, 20)
  line L14 (-41.8787, 20) -> (-31, 20)
  line L15 (-31, 20) -> (-31, 26)
  circle A3 centre (36, -14.5) radius 1.9
  arc A4 (-38.922, -26.9266) -> (-34.8649, -28.3108) centre (-36, -25) ccw
  line L16 (-34.8649, -28.3108) -> (-32.5, -27.5)
  line L17 (-32.5, -27.5) -> (32.5, -27.5)
  line L18 (32.5, -27.5) -> (32.5, -19)
  arc A5 (33.5, -18) -> (32.5, -19) centre (33.5, -19) ccw
  line L19 (33.5, -18) -> (38.5, -18)
  arc A6 (38.5, -18) -> (39.5, -17) centre (38.5, -17) ccw
  line L20 (39.5, -17) -> (39.5, -12)
  arc A7 (40.5, -11) -> (39.5, -12) centre (40.5, -12) ccw
  line L21 (40.5, -11) -> (56.5, -11)
  line L22 (56.5, -11) -> (56.5, 11)
  line L23 (56.5, 11) -> (40.5, 11)
  arc A8 (39.5, 12) -> (40.5, 11) centre (40.5, 12) ccw
  line L24 (39.5, 12) -> (39.5, 17)
  arc A9 (39.5, 17) -> (38.5, 18) centre (38.5, 17) ccw
  line L25 (38.5, 18) -> (33.5, 18)
  arc A10 (32.5, 19) -> (33.5, 18) centre (33.5, 19) ccw
  line L26 (32.5, 19) -> (32.5, 27.5)
  line L27 (32.5, 27.5) -> (-32.5, 27.5)
  line L28 (-32.5, 27.5) -> (-34.8649, 28.3108)
  arc A11 (-34.8649, 28.3108) -> (-38.922, 26.9266) centre (-36, 25) ccw
  line L29 (-38.922, 26.9266) -> (-42.5, 21.5)
  line L30 (-42.5, 21.5) -> (-57.5, 6.5)
  line L31 (-57.5, 6.5) -> (-57.5, -6.5)
  line L32 (-57.5, -6.5) -> (-42.5, -21.5)
  line L33 (-42.5, -21.5) -> (-38.922, -26.9266)
  line L34 (32.5, -19) -> (31, -19)
  line L35 (32.5, 19) -> (31, 19)
  constraint coincident L18.end A5.end
  constraint coincident L5 L34.end
  constraint coincident A10.start L26.start
  constraint coincident L1 L35.end
extrude "Extrusion21" add sketch "Skizze23" along normal blind 5.5 contours L0 L1 L5 L6 L7 L8 L9 L10 L11 L12 L13 L14 L15 A4 L16 L17 L18 L26 L27 L28 A11 L29 L30 L31 L32 L33 L34 L35 bodies 2
sketch "Skizze24" plane through (56.5, 0, 0) normal (1, 0, 0) x (0, 0, -1)
  line L0 (-11, 21.5) -> (11, 21.5)
  line L1 (11, 21.5) -> (11, 45)
  line L2 (11, 45) -> (-11, 45)
  line L3 (-11, 45) -> (-11, 21.5)
  circle A0 centre (0, 21.5) radius 5
  dimension "d114" = 10
  constraint midpoint L0 A0.centre
  measures "d114" diameter of A0
extrude "Extrusion22" cut sketch "Skizze24" against normal blind 5 contours L0 A0 picked at (1.2218, 23.6161) bodies 2
sketch "Skizze25" plane through (-57.5, 0, 0) normal (-1, 0, 0) x (0, 0, 1)
  line L0 (6.5, 16) -> (6.5, 45)
  line L1 (6.5, 45) -> (-6.5, 45)
  line L2 (-6.5, 45) -> (-6.5, 16)
  line L3 (-6.5, 16) -> (6.5, 16)
  circle A0 centre (0, 16) radius 5
  dimension "d117" = 10
  constraint midpoint L3 A0.centre
  measures "d117" diameter of A0
extrude "Extrusion23" cut sketch "Skizze25" against normal blind 6 contours L3 A0 picked at (1.4325, 17.6785) bodies 2
sketch "Skizze26" plane through (0, 0, 27.5) normal (0, 0, 1) x (1, 0, 0)
  line L0 (32.5, 16) -> (32.5, 45)
  line L1 (32.5, 45) -> (-32.5, 45)
  line L2 (-32.5, 45) -> (-32.5, 16)
  line L3 (-32.5, 16) -> (32.5, 16)
  line L4 (22.5, 45) -> (10.5, 45)
  line L5 (10.5, 45) -> (10.5, 37)
  line L6 (10.5, 37) -> (22.5, 37)
  line L7 (22.5, 37) -> (22.5, 45)
  dimension "d120" = 10
  dimension "d121" = 21
  dimension "d122" = 12
  constraint horizontal L4
  constraint vertical L5
  constraint horizontal L6
  constraint vertical L7
  constraint coincident L1 L4.start
  measures "d120" distance of L0 L7
  measures "d121" distance of L3 L6
  measures "d122" horizontal distance of L5.end L6.end
extrude "Extrusion24" cut sketch "Skizze26" against normal blind 2 contours L1 L4 L5 L6 L7 bodies 2
sketch "Skizze27" plane through (0, 45, 0) normal (0, 1, 0) x (-1, 0, 0)
  line L0 (-22.5, 26) -> (-22.5, 27.5)
  line L1 (-22.5, 27.5) -> (-32.5, 27.5)
  line L2 (-32.5, 27.5) -> (-32.5, 19)
  arc A0 (-33.5, 18) -> (-32.5, 19) centre (-33.5, 19) ccw
  line L3 (-33.5, 18) -> (-38.5, 18)
  arc A1 (-38.5, 18) -> (-39.5, 17) centre (-38.5, 17) ccw
  line L4 (-39.5, 17) -> (-39.5, 12)
  arc A2 (-40.5, 11) -> (-39.5, 12) centre (-40.5, 12) ccw
  line L5 (-40.5, 11) -> (-56.5, 11)
  line L6 (-56.5, 11) -> (-56.5, -11)
  line L7 (-56.5, -11) -> (-40.5, -11)
  arc A3 (-39.5, -12) -> (-40.5, -11) centre (-40.5, -12) ccw
  line L8 (-39.5, -12) -> (-39.5, -17)
  arc A4 (-39.5, -17) -> (-38.5, -18) centre (-38.5, -17) ccw
  line L9 (-38.5, -18) -> (-33.5, -18)
  arc A5 (-32.5, -19) -> (-33.5, -18) centre (-33.5, -19) ccw
  line L10 (-32.5, -19) -> (-32.5, -27.5)
  line L11 (-32.5, -27.5) -> (32.5, -27.5)
  line L12 (32.5, -27.5) -> (34.8649, -28.3108)
  arc A6 (34.8649, -28.3108) -> (38.922, -26.9266) centre (36, -25) ccw
  line L13 (38.922, -26.9266) -> (42.5, -21.5)
  line L14 (42.5, -21.5) -> (57.5, -6.5)
  line L15 (57.5, -6.5) -> (57.5, 6.5)
  line L16 (57.5, 6.5) -> (42.5, 21.5)
  line L17 (42.5, 21.5) -> (38.922, 26.9266)
  arc A7 (38.922, 26.9266) -> (34.8649, 28.3108) centre (36, 25) ccw
  line L18 (34.8649, 28.3108) -> (32.5, 27.5)
  line L19 (32.5, 27.5) -> (-10.5, 27.5)
  line L20 (-10.5, 27.5) -> (-10.5, 26)
  line L21 (-10.5, 26) -> (31, 26)
  line L22 (31, 26) -> (31, 20)
  line L23 (31, 20) -> (41.8787, 20)
  line L24 (41.8787, 20) -> (51.5218, 10.3569)
  line L25 (51.5218, 10.3569) -> (51.5218, -10.3569)
  line L26 (51.5218, -10.3569) -> (41.8787, -20)
  line L27 (41.8787, -20) -> (31, -20)
  line L28 (31, -20) -> (31, -26)
  line L29 (31, -26) -> (23, -26)
  line L30 (23, -26) -> (-23, -26)
  line L31 (-23, -26) -> (-31, -26)
  line L32 (-31, -26) -> (-31, -9.5)
  line L33 (-31, -9.5) -> (-51.5, -9.5)
  line L34 (-51.5, -9.5) -> (-51.5, 9.5)
  line L35 (-51.5, 9.5) -> (-31, 9.5)
  line L36 (-31, 9.5) -> (-31, 26)
  line L37 (-31, 26) -> (-22.5, 26)
  circle A8 centre (-36, -14.5) radius 1.9
  circle A9 centre (36, -25) radius 1.9
  circle A10 centre (36, 25) radius 1.9
  circle A11 centre (-36, 14.5) radius 1.9
  line L38 (-22.5, 26) -> (-10.5, 26)
  line L39 (-10.5, 26) -> (-10.5, 27.5)
  line L40 (-10.5, 27.5) -> (-22.5, 27.5)
  line L41 (-22.5, 27.5) -> (-22.5, 26)
extrude "Extrusion25" add sketch "Skizze27" along normal blind 2 contours L0 L1 L2 A0 L3 A1 L4 A2 L5 L6 L7 A3 L8 A4 L9 A5 L10 L11 L12 A6 L13 L14 L15 L16 L17 A7 L18 L19 L20 L21 L22 L23 L24 L25 L26 L27 L28 L29 L30 L31 L32 L33 L34 L35 L36 L37 L39 L41 | L21 L22 L23 L24 L25 L26 L27 L28 L29 L30 L31 L32 L33 L34 L35 L36 L37 L38 bodies 2
extrude "Extrusion26" cut 1 faces at (14.5, 46.3333, 26) along direction (0, 0, -1) blind 4.5 on bodies 2 bodies 2
sketch "Skizze28" plane through (0, 47, 0) normal (0, 1, 0) x (-1, 0, 0)
  line L0 (-22.5, 21.5) -> (-22.5, 27.5)
  line L1 (-22.5, 27.5) -> (-32.5, 27.5)
  line L2 (-32.5, 27.5) -> (-32.5, 19)
  arc A0 (-33.5, 18) -> (-32.5, 19) centre (-33.5, 19) ccw
  line L3 (-33.5, 18) -> (-38.5, 18)
  arc A1 (-38.5, 18) -> (-39.5, 17) centre (-38.5, 17) ccw
  line L4 (-39.5, 17) -> (-39.5, 12)
  arc A2 (-40.5, 11) -> (-39.5, 12) centre (-40.5, 12) ccw
  line L5 (-40.5, 11) -> (-56.5, 11)
  line L6 (-56.5, 11) -> (-56.5, -11)
  line L7 (-56.5, -11) -> (-40.5, -11)
  arc A3 (-39.5, -12) -> (-40.5, -11) centre (-40.5, -12) ccw
  line L8 (-39.5, -12) -> (-39.5, -17)
  arc A4 (-39.5, -17) -> (-38.5, -18) centre (-38.5, -17) ccw
  line L9 (-38.5, -18) -> (-33.5, -18)
  arc A5 (-32.5, -19) -> (-33.5, -18) centre (-33.5, -19) ccw
  line L10 (-32.5, -19) -> (-32.5, -27.5)
  line L11 (-32.5, -27.5) -> (32.5, -27.5)
  line L12 (32.5, -27.5) -> (34.8649, -28.3108)
  arc A6 (34.8649, -28.3108) -> (38.922, -26.9266) centre (36, -25) ccw
  line L13 (38.922, -26.9266) -> (42.5, -21.5)
  line L14 (42.5, -21.5) -> (57.5, -6.5)
  line L15 (57.5, -6.5) -> (57.5, 6.5)
  line L16 (57.5, 6.5) -> (42.5, 21.5)
  line L17 (42.5, 21.5) -> (38.922, 26.9266)
  arc A7 (38.922, 26.9266) -> (34.8649, 28.3108) centre (36, 25) ccw
  line L18 (34.8649, 28.3108) -> (32.5, 27.5)
  line L19 (32.5, 27.5) -> (-10.5, 27.5)
  line L20 (-10.5, 27.5) -> (-10.5, 21.5)
  line L21 (-10.5, 21.5) -> (-22.5, 21.5)
  circle A8 centre (-36, 14.5) radius 1.9
  circle A9 centre (36, -25) radius 1.9
  circle A10 centre (-36, -14.5) radius 1.9
  circle A11 centre (36, 25) radius 1.9
  circle A12 centre (3.5, 16) radius 6.5
  dimension "d129" = 36
  dimension "d130" = 13
  dimension "d131" = 11.5
  measures "d129" distance of L2 A12.centre
  measures "d130" diameter of A12
  measures "d131" distance of L19 A12.centre
extrude "Extrusion27" cut sketch "Skizze28" against normal blind 2 contours A12 bodies 2
sketch "Skizze29" plane through (0, 47, 0) normal (0, 1, 0) x (-1, 0, 0)
  circle A0 centre (3.5, 16) radius 6.5
  line L0 (-22.5, 21.5) -> (-22.5, 27.5)
  line L1 (-22.5, 27.5) -> (-32.5, 27.5)
  line L2 (-32.5, 27.5) -> (-32.5, 19)
  arc A1 (-33.5, 18) -> (-32.5, 19) centre (-33.5, 19) ccw
  line L3 (-33.5, 18) -> (-38.5, 18)
  arc A2 (-38.5, 18) -> (-39.5, 17) centre (-38.5, 17) ccw
  line L4 (-39.5, 17) -> (-39.5, 12)
  arc A3 (-40.5, 11) -> (-39.5, 12) centre (-40.5, 12) ccw
  line L5 (-40.5, 11) -> (-56.5, 11)
  line L6 (-56.5, 11) -> (-56.5, -11)
  line L7 (-56.5, -11) -> (-40.5, -11)
  arc A4 (-39.5, -12) -> (-40.5, -11) centre (-40.5, -12) ccw
  line L8 (-39.5, -12) -> (-39.5, -17)
  arc A5 (-39.5, -17) -> (-38.5, -18) centre (-38.5, -17) ccw
  line L9 (-38.5, -18) -> (-33.5, -18)
  arc A6 (-32.5, -19) -> (-33.5, -18) centre (-33.5, -19) ccw
  line L10 (-32.5, -19) -> (-32.5, -27.5)
  line L11 (-32.5, -27.5) -> (32.5, -27.5)
  line L12 (32.5, -27.5) -> (34.8649, -28.3108)
  arc A7 (34.8649, -28.3108) -> (38.922, -26.9266) centre (36, -25) ccw
  line L13 (38.922, -26.9266) -> (42.5, -21.5)
  line L14 (42.5, -21.5) -> (57.5, -6.5)
  line L15 (57.5, -6.5) -> (57.5, 6.5)
  line L16 (57.5, 6.5) -> (42.5, 21.5)
  line L17 (42.5, 21.5) -> (38.922, 26.9266)
  arc A8 (38.922, 26.9266) -> (34.8649, 28.3108) centre (36, 25) ccw
  line L18 (34.8649, 28.3108) -> (32.5, 27.5)
  line L19 (32.5, 27.5) -> (-10.5, 27.5)
  line L20 (-10.5, 27.5) -> (-10.5, 21.5)
  line L21 (-10.5, 21.5) -> (-22.5, 21.5)
  circle A9 centre (-36, 14.5) radius 1.9
  circle A10 centre (36, -25) radius 1.9
  circle A11 centre (-36, -14.5) radius 1.9
  circle A12 centre (36, 25) radius 1.9
  line L22 (21.5, -4.5) -> (-5.5, -4.5)
  line L23 (-5.5, -4.5) -> (-5.5, -20.5)
  line L24 (-5.5, -20.5) -> (21.5, -20.5)
  line L25 (21.5, -20.5) -> (21.5, -4.5)
  dimension "d134" = 27
  dimension "d135" = 27
  dimension "d136" = 16
  dimension "d137" = 7
  constraint horizontal L22
  constraint vertical L23
  constraint horizontal L24
  constraint vertical L25
  measures "d134" distance of L10 L23
  measures "d135" horizontal distance of L22.start L22.end
  measures "d136" vertical distance of L22.start L24.end
  measures "d137" distance of L11 L24
extrude "Extrusion28" cut sketch "Skizze29" against normal blind 2 contours L22 L23 L24 L25 bodies 2
sketch "Skizze30" plane through (0, 0, 27.5) normal (0, 0, 1) x (1, 0, 0)
  line L0 (22.5, 47) -> (22.5, 37)
  line L1 (22.5, 37) -> (10.5, 37)
  line L2 (10.5, 37) -> (10.5, 47)
  line L3 (10.5, 47) -> (-32.5, 47)
  line L4 (-32.5, 47) -> (-32.5, 16)
  line L5 (-32.5, 16) -> (32.5, 16)
  line L6 (32.5, 16) -> (32.5, 47)
  line L7 (32.5, 47) -> (22.5, 47)
  line L8 (28.6326, 22.8418) -> (18.6326, 34.8418)
  arc A0 (18.6326, 34.8418) -> (16.3279, 32.9212) centre (17.4802, 33.8815) ccw
  line L9 (16.3279, 32.9212) -> (26.3279, 20.9212)
  arc A1 (26.3279, 20.9212) -> (28.6326, 22.8418) centre (27.4802, 21.8815) ccw
  line L10 (27.4802, 21.8815) -> (17.4802, 33.8815) construction
  line L11 (7.1279, 32.9212) -> (17.1279, 20.9212)
  arc A2 (9.4326, 34.8418) -> (7.1279, 32.9212) centre (8.2802, 33.8815) ccw
  line L12 (19.4326, 22.8418) -> (9.4326, 34.8418)
  arc A3 (17.1279, 20.9212) -> (19.4326, 22.8418) centre (18.2802, 21.8815) ccw
  line L13 (-2.0721, 32.9212) -> (7.9279, 20.9212)
  arc A4 (0.2326, 34.8418) -> (-2.0721, 32.9212) centre (-0.9198, 33.8815) ccw
  line L14 (10.2326, 22.8418) -> (0.2326, 34.8418)
  arc A5 (7.9279, 20.9212) -> (10.2326, 22.8418) centre (9.0802, 21.8815) ccw
  line L15 (-11.2721, 32.9212) -> (-1.2721, 20.9212)
  arc A6 (-8.9674, 34.8418) -> (-11.2721, 32.9212) centre (-10.1198, 33.8815) ccw
  line L16 (1.0326, 22.8418) -> (-8.9674, 34.8418)
  arc A7 (-1.2721, 20.9212) -> (1.0326, 22.8418) centre (-0.1198, 21.8815) ccw
  line L17 (-20.4721, 32.9212) -> (-10.4721, 20.9212)
  arc A8 (-18.1674, 34.8418) -> (-20.4721, 32.9212) centre (-19.3198, 33.8815) ccw
  line L18 (-8.1674, 22.8418) -> (-18.1674, 34.8418)
  arc A9 (-10.4721, 20.9212) -> (-8.1674, 22.8418) centre (-9.3198, 21.8815) ccw
  line L19 (-29.6721, 32.9212) -> (-19.6721, 20.9212)
  arc A10 (-27.3674, 34.8418) -> (-29.6721, 32.9212) centre (-28.5198, 33.8815) ccw
  line L20 (-17.3674, 22.8418) -> (-27.3674, 34.8418)
  arc A11 (-19.6721, 20.9212) -> (-17.3674, 22.8418) centre (-18.5198, 21.8815) ccw
  dimension "d140" = 3
  dimension "d143" = -46
  dimension "d144" = 0
  constraint tangent L8 A0
  constraint tangent A0 L9
  constraint parallel L8 L9
  constraint tangent L9 A1
  constraint tangent L8 A1
  measures "d140" diameter of A0
extrude "Extrusion29" cut sketch "Skizze30" against normal blind 2 contours L8 A0 L9 A1 | L11 A2 L12 A3 | L13 A4 L14 A5 | L15 A6 L16 A7 | L17 A8 L18 A9 | L19 A10 L20 A11 bodies 2
sketch "Skizze31" plane through (0, 47, 0) normal (0, 1, 0) x (-1, 0, 0)
  line L0 (-5.5, -4.5) -> (21.5, -4.5)
  line L1 (21.5, -4.5) -> (21.5, -20.5)
  line L2 (21.5, -20.5) -> (-5.5, -20.5)
  line L3 (-5.5, -20.5) -> (-5.5, -4.5)
  circle A0 centre (3.5, 16) radius 6.5
  line L4 (-22.5, 21.5) -> (-22.5, 27.5)
  line L5 (-22.5, 27.5) -> (-32.5, 27.5)
  line L6 (-32.5, 27.5) -> (-32.5, 19)
  arc A1 (-33.5, 18) -> (-32.5, 19) centre (-33.5, 19) ccw
  line L7 (-33.5, 18) -> (-38.5, 18)
  arc A2 (-38.5, 18) -> (-39.5, 17) centre (-38.5, 17) ccw
  line L8 (-39.5, 17) -> (-39.5, 12)
  arc A3 (-40.5, 11) -> (-39.5, 12) centre (-40.5, 12) ccw
  line L9 (-40.5, 11) -> (-56.5, 11)
  line L10 (-56.5, 11) -> (-56.5, -11)
  line L11 (-56.5, -11) -> (-40.5, -11)
  arc A4 (-39.5, -12) -> (-40.5, -11) centre (-40.5, -12) ccw
  line L12 (-39.5, -12) -> (-39.5, -17)
  arc A5 (-39.5, -17) -> (-38.5, -18) centre (-38.5, -17) ccw
  line L13 (-38.5, -18) -> (-33.5, -18)
  arc A6 (-32.5, -19) -> (-33.5, -18) centre (-33.5, -19) ccw
  line L14 (-32.5, -19) -> (-32.5, -27.5)
  line L15 (-32.5, -27.5) -> (32.5, -27.5)
  line L16 (32.5, -27.5) -> (34.8649, -28.3108)
  arc A7 (34.8649, -28.3108) -> (38.922, -26.9266) centre (36, -25) ccw
  line L17 (38.922, -26.9266) -> (42.5, -21.5)
  line L18 (42.5, -21.5) -> (57.5, -6.5)
  line L19 (57.5, -6.5) -> (57.5, 6.5)
  line L20 (57.5, 6.5) -> (42.5, 21.5)
  line L21 (42.5, 21.5) -> (38.922, 26.9266)
  arc A8 (38.922, 26.9266) -> (34.8649, 28.3108) centre (36, 25) ccw
  line L22 (34.8649, 28.3108) -> (32.5, 27.5)
  line L23 (32.5, 27.5) -> (-10.5, 27.5)
  line L24 (-10.5, 27.5) -> (-10.5, 21.5)
  line L25 (-10.5, 21.5) -> (-22.5, 21.5)
  circle A9 centre (-36, 14.5) radius 1.9
  circle A10 centre (36, 25) radius 1.9
  circle A11 centre (-36, -14.5) radius 1.9
  circle A12 centre (36, -25) radius 1.9
  line L26 (21.5, -4.5) -> (-5.5, -4.5)
  line L27 (-5.5, -4.5) -> (-5.5, -20.5)
  line L28 (-5.5, -20.5) -> (21.5, -20.5)
  line L29 (21.5, -20.5) -> (21.5, -4.5)
  circle A13 centre (3.5, 16) radius 6.5
  line L30 (-22.5, 26) -> (-22.5, 21.5)
  line L31 (-22.5, 21.5) -> (-10.5, 21.5)
  line L32 (-10.5, 21.5) -> (-10.5, 26)
  line L33 (-10.5, 26) -> (31, 26)
  line L34 (31, 26) -> (31, 20)
  line L35 (31, 20) -> (41.8787, 20)
  line L36 (41.8787, 20) -> (51.5218, 10.3569)
  line L37 (51.5218, 10.3569) -> (51.5218, -10.3569)
  line L38 (51.5218, -10.3569) -> (41.8787, -20)
  line L39 (41.8787, -20) -> (31, -20)
  line L40 (31, -20) -> (31, -26)
  line L41 (31, -26) -> (23, -26)
  line L42 (23, -26) -> (-23, -26)
  line L43 (-23, -26) -> (-31, -26)
  line L44 (-31, -26) -> (-31, -9.5)
  line L45 (-31, -9.5) -> (-51.5, -9.5)
  line L46 (-51.5, -9.5) -> (-51.5, 9.5)
  line L47 (-51.5, 9.5) -> (-31, 9.5)
  line L48 (-31, 9.5) -> (-31, 26)
  line L49 (-31, 26) -> (-22.5, 26)
  line L50 (-12, 21.5) -> (-21, 21.5)
  line L51 (-21, 21.5) -> (-21, 11.5)
  line L52 (-21, 11.5) -> (-12, 11.5)
  line L53 (-12, 11.5) -> (-12, 21.5)
  dimension "d147" = 9
  dimension "d148" = 10
  dimension "d149" = 11
  dimension "d151" = 1.5
  constraint horizontal L50
  constraint vertical L51
  constraint horizontal L52
  constraint vertical L53
  constraint coincident L25 L50.start
  measures "d147" distance of L50.start L50.end
  measures "d148" distance of L50.start L52.end
  measures "d151" distance of L24 L53
extrude "Extrusion30" cut sketch "Skizze31" against normal blind 2 contours L25 L31 L50 L51 L52 L53 bodies 2
chamfer "Fase1" distance 3 distance2 2 2 edges at (-8, 47, -20.5) (-8, 47, -4.5) measured on face at (-40.5, 47, 7.8333) measured on face at (-40.5, 47, 7.8333) on bodies 2